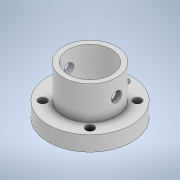
# Autodesk Inventor part: Brida para herramienta
Saved by Autodesk Inventor 2022 (Build 260153000, 153)
## iProperties
Created: 2022-08-23
Part Number: Brida para herramienta
Material: Generic
Document SubType Name: Modeling
Designer: David
Density: 1 g/cm^3
Appearance: Default
Author: David
Autodesk Inventor part; units mm, degrees
ref_plane "XZ Plane" through (0, 0, 0) normal (0, 1, 0) x (-1, 0, 0)
ref_plane "XY Plane" through (0, 0, 0) normal (0, 0, 1) x (1, 0, 0)
sketch "Sketch1" plane through (0, 0, 0) normal (0, 1, 0) x (-1, 0, 0)
  circle A0 centre (0, 0) radius 25
  dimension "d0" = 50
  constraints: 1 centre point, 1 coincident
  measures "d0" diameter of A0
extrude "Extrusion1" add sketch "Sketch1" along normal blind 9
sketch "Sketch2" plane through (0, 0, 0) normal (0, -1, 0) x (1, 0, 0)
  circle A0 centre (0, 0) radius 12.5
  dimension "d3" = 25
  constraints: 1 centre point, 1 coincident
  measures "d3" diameter of A0
extrude "Extrusion2" cut sketch "Sketch2" against normal blind 6
sketch "Sketch3" plane through (0, 9, 0) normal (0, 1, 0) x (1, 0, 0)
  circle A0 centre (0, 0) radius 20
  line L0 (0, 35) -> (0, -35) projected
  line L1 (0, 0) -> (14.1421, 14.1421)
  line L2 (-35, 0) -> (35, 0) projected
  point P0 (0, 20)
  dimension "d6" = 40
  dimension "d15" = 45
  constraints: 2 coincident, 2 end point, 2 point on circle, 1 centre point, 1 point on line
  measures "d6" diameter of A0
  measures "d15" angle of L2 L1
hole "Hole1" at (0, 9, -20) direction (0, -1, 0) diameter 6 end through all
hole "Hole2" at (14.1421, 9, -14.1421) direction (0, -1, 0) diameter 4.917 end through all thread size "M6x1" class "6H" standard "ISO Metric profile"
pattern_circular "Circular Pattern1" count 4 over 360 about axis through (0, 0, 0) along (0, 1, 0) of "Hole2"
sketch "Sketch8" plane through (0, 9, 0) normal (0, 1, 0) x (1, 0, 0)
  circle A0 centre (0, 0) radius 16
  dimension "d49" = 32
  constraints: 1 centre point, 1 coincident
  measures "d49" diameter of A0
extrude "Extrusion5" add sketch "Sketch8" along normal blind 20
ref_plane "Work Plane1" through (16, 9, 0) normal (1, 0, 0) x (0, 1, 0)
sketch "Sketch15" plane through (16, 9, 0) normal (1, 0, 0) x (0, 1, 0)
  line L0 (0, -16) -> (20, -16) projected
  line L1 (20, -16) -> (20, 16) projected
  line L2 (-14.8, 0) -> (25.8, 0) projected
  point P0 (-9, 0)
  point P1 (10, 0)
  dimension "d60" = 10
  dimension "d61" = 20
  constraints: 1 point on line
  measures "d60" distance from line of L1 point (10, 0)
  measures "d61" distance of L0.start L0.end
hole "Hole4" at (16, 19, 0) direction (-1, 0, 0) diameter 6 end through all
sketch "Sketch16" plane through (0, 29, 0) normal (0, 1, 0) x (1, 0, 0)
  circle A0 centre (0, 0) radius 13
  circle A1 centre (0, 0) radius 16 projected
  dimension "d70" = 3
  constraints: 1 centre point, 1 coincident
  measures "d70" radial gap between concentric circles of A0 A1
extrude "Extrusion7" cut sketch "Sketch16" against normal up to surface (20 mm away) contours A0
equation "\"d60\" = 0.5 * d61"
body "Solid1"
